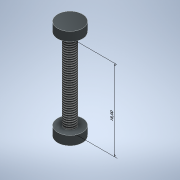
# Autodesk Inventor part: servo-hotn-bolt
Saved by Autodesk Inventor 2021 (Build 250183000, 183)
## iProperties
Created: 2021-02-27
Part Number: servo-hotn-bolt
Material: Iron, Ductile
Document SubType Name: Modeling
Designer: WASHINGTON
Density: 7.15 g/cm^3
Appearance: Iron Gray
Author: WASHINGTON
Autodesk Inventor part; units mm, degrees
ref_plane "YZ Plane" through (0, 0, 0) normal (1, 0, 0) x (0, 1, 0)
ref_plane "XZ Plane" through (0, 0, 0) normal (0, 1, 0) x (-1, 0, 0)
ref_plane "XY Plane" through (0, 0, 0) normal (0, 0, 1) x (1, 0, 0)
sketch "Sketch1" plane through (0, 0, 0) normal (1, 0, 0) x (0, 1, 0)
  line L0 (0, 0) -> (0, 2.75)
  line L1 (0, 2.75) -> (2, 2.75)
  line L2 (2, 2.75) -> (2, 1.25)
  line L3 (2, 1.25) -> (20, 1.25)
  line L4 (20, 1.25) -> (20, 2.75)
  line L5 (20, 2.75) -> (22, 2.75)
  line L6 (22, 2.75) -> (22, 0)
  line L7 (22, 0) -> (0, 0)
  dimension "d0" = 2
  dimension "d1" = 2
  dimension "d3" = 1.25
  dimension "d4" = 1.5
  dimension "d5" = 18
  constraints: 16 end point, 6 perpendicular, 2 point on line, 1 vertical
  measures "d0" distance of L4.end L5.end
  measures "d1" distance of L0.end L1.end
  measures "d3" distance from line of L0.start L3
  measures "d4" distance of L3.end L4.end
  measures "d5" distance of L2.end L3.end
revolve "Revolution1" add sketch "Sketch1" angle 360 about axis through (0, 22, 0) along (0, -1, 0)
thread "Thread1" size "M2.5x0.45" class "6g" standard "ANSI Metric M Profile" full length
body "Solid1"
